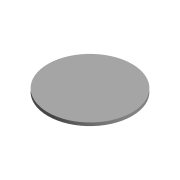
# Autodesk Inventor part: encoder_wheel
Saved by Autodesk Inventor 2014 (Build 180170000, 170)
## iProperties
Created: 2014-01-08
Part Number: encoder_wheel
Material: Generisch
Document SubType Name: Modeling
Designer: Felix
Density: 1 g/cm^3
Appearance: Vorgabe
Author: Felix
Autodesk Inventor part; units mm, degrees
ref_plane "YZ Plane" through (0, 0, 0) normal (1, 0, 0) x (0, 1, 0)
ref_plane "XZ Plane" through (0, 0, 0) normal (0, 1, 0) x (-1, 0, 0)
sketch "Skizze1" plane through (0, 0, 0) normal (0, 0, 1) x (1, 0, 0)
  circle A0 centre (0, 0) radius 23.3 projected
  circle A1 centre (0, 0) radius 22.8
  point P0 (0, 0)
  dimension "d0" = 0.5
  constraints: 1 centre point, 1 coincident
  measures "d0" radial gap between concentric circles of A1 A0
ref_plane "Arbeitsebene1" through (-8.8685, -8.875, -1.7) normal (0, 0, 1) x (1, 0, 0)
extrude "Extrusion1" add sketch "Skizze1" against normal up to surface (1.7 mm away) contours A1
